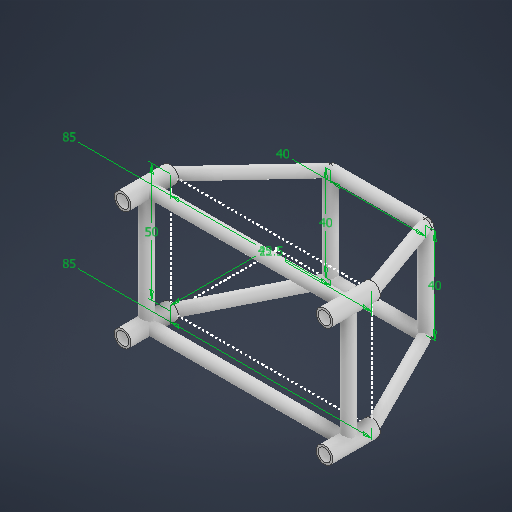
# Autodesk Inventor part: RCPlaneSkeletonFrontFront1
Saved by Autodesk Inventor 2026.1 (Build 301233000, 233)
## iProperties
Created: 2026-03-11
Part Number: RCPlaneSkeletonFrontFront1
Material: Generic
Document SubType Name: Modeling
Designer: morri
Density: 1 g/cm^3
Appearance: Default
Author: morri
Autodesk Inventor part; units mm, degrees
ref_plane "YZ Plane" through (0, 0, 0) normal (1, 0, 0) x (0, 1, 0)
sketch "Sketch1" plane through (0, 0, 0) normal (0, 0, 1) x (1, 0, 0)
  circle A0 centre (0, 0) radius 2.5
  circle A1 centre (0, 50) radius 2.5
  circle A2 centre (85, 50) radius 2.5
  circle A3 centre (85, 0) radius 2.5
  dimension "d10" = 5
  dimension "d11" = 5
  dimension "d12" = 5
  dimension "d13" = 5
  constraints: 4 centre point, 1 coincident
  measures "d10" diameter of A0
  measures "d11" diameter of A1
  measures "d12" diameter of A2
  measures "d13" diameter of A3
sketch3d "3D Sketch1"
  line L0 (85, 50, 0) -> (62.5, 40, -45)
  dimension "d0" = 45
  dimension "d1" = 22.5
  dimension "d2" = 40
  dimension "d3" = 40
  dimension "d4" = 40
  dimension "d5" = 85
  dimension "d6" = 50
  dimension "d7" = 85
sweep "Sweep1" add profiles "Sketch1" path "3D Sketch1" contours A2
sketch3d "3D Sketch1 for Sweep2"
  line L0 (0, 50, 0) -> (22.5, 40, -45)
  dimension "d0" = 45
  dimension "d1" = 22.5
  dimension "d2" = 40
  dimension "d3" = 40
  dimension "d4" = 40
  dimension "d5" = 85
  dimension "d6" = 50
  dimension "d7" = 85
sweep "Sweep2" add profiles "Sketch1" path "3D Sketch1 for Sweep2" separate body contours A1
sketch3d "3D Sketch1 for Sweep3"
  line L0 (0, 0, 0) -> (22.5, 0, -45)
  dimension "d0" = 45
  dimension "d1" = 22.5
  dimension "d2" = 40
  dimension "d3" = 40
  dimension "d4" = 40
  dimension "d5" = 85
  dimension "d6" = 50
  dimension "d7" = 85
sweep "Sweep3" add profiles "Sketch1" path "3D Sketch1 for Sweep3" separate body contours A0
sketch3d "3D Sketch1 for Sweep4"
  line L0 (85, 0, 0) -> (62.5, 0, -45)
  dimension "d0" = 45
  dimension "d1" = 22.5
  dimension "d2" = 40
  dimension "d3" = 40
  dimension "d4" = 40
  dimension "d5" = 85
  dimension "d6" = 50
  dimension "d7" = 85
sweep "Sweep4" add profiles "Sketch1" path "3D Sketch1 for Sweep4" separate body contours A3
ref_plane "Work Plane1" through (0, 0, 0) normal (0, 1, 0) x (-1, 0, 0)
sketch "Sketch2" plane through (0, 0, 0) normal (0, 1, 0) x (-1, 0, 0)
  line L0 (-65, -45) -> (-60, -45) projected
  circle A0 centre (-62.5, -45) radius 2.5
  line L1 (-25, -45) -> (-20, -45) projected
  circle A1 centre (-22.5, -45) radius 2.5
  point P0 (0, 0)
  dimension "d24" = 5
  dimension "d25" = 5
  constraints: 2 centre point, 2 midpoint
  measures "d24" diameter of A0
  measures "d25" diameter of A1
extrude "Extrusion2" add sketch "Sketch2" along normal blind 40 separate body
ref_plane "Work Plane3" through (22.5, 0, -45) normal (-1, 0, 0) x (0, -1, 0)
sketch "Sketch4" plane through (22.5, 0, -45) normal (-1, 0, 0) x (0, -1, 0)
  line L0 (0, 2.5) -> (0, -2.5) projected
  circle A0 centre (0, 0) radius 2.5
  line L1 (-42.5, 0) -> (-37.5, 0) projected
  circle A1 centre (-40, 0) radius 2.5
  point P0 (0, 45)
  dimension "d36" = 5
  dimension "d37" = 5
  constraints: 2 centre point, 2 midpoint
  measures "d36" diameter of A0
  measures "d37" diameter of A1
extrude "Extrusion4" add sketch "Sketch4" against normal blind 40 separate body
sketch "Sketch10" plane through (0, 0, 0) normal (0, 0, 1) x (1, 0, 0)
  circle A0 centre (0, 0) radius 3.5
  circle A1 centre (0, 50) radius 2.5 construction
  circle A2 centre (0, 50) radius 3.5
  circle A3 centre (85, 50) radius 2.5 construction
  circle A4 centre (85, 50) radius 3.5
  circle A5 centre (85, 0) radius 2.5 construction
  circle A6 centre (85, 0) radius 3.5
  dimension "d69" = 7
  dimension "d70" = 7
  dimension "d71" = 7
  dimension "d72" = 7
  constraints: 4 centre point, 4 coincident
  measures "d69" diameter of A0
  measures "d70" diameter of A2
  measures "d71" diameter of A4
  measures "d72" diameter of A6
extrude "Extrusion8" add sketch "Sketch10" along normal blind 20 separate body
sketch "Sketch11" plane through (0, 0, 0) normal (0, 1, 0) x (-1, 0, 0)
  line L0 (0, 0) -> (0, 10) construction
  line L1 (0, 0) -> (-85, 0) construction
  line L2 (-85, 0) -> (-85, 10) construction
  line L3 (-85, 10) -> (0, 10) construction
  line L4 (0, 10) -> (0, 0) construction
  circle A0 centre (0, 10) radius 2.5
  circle A1 centre (-85, 10) radius 2.5
  dimension "d77" = 85
  dimension "d78" = 5
  dimension "d79" = 5
  constraints: 10 end point, 2 centre point, 2 coincident, 2 parallel, 1 horizontal, 1 perpendicular, 1 vertical
  measures "d77" distance of L2.end L3.end
  measures "d78" diameter of A0
  measures "d79" diameter of A1
extrude "Extrusion9" add sketch "Sketch11" along normal blind 50 separate body
sketch "Sketch12" plane through (0, 0, 0) normal (1, 0, 0) x (0, 1, 0)
  circle A0 centre (0, 10) radius 2.5
  line L0 (50, 7.5) -> (50, 12.5) construction
  circle A1 centre (50, 10) radius 2.5
  point P0 (0, 0)
  dimension "d82" = 5
  dimension "d83" = 5
  constraints: 2 centre point, 1 midpoint
  measures "d82" diameter of A0
  measures "d83" diameter of A1
extrude "Extrusion10" add sketch "Sketch12" along normal blind 85 separate body
sketch "Sketch13" plane through (0, 0, 20) normal (0, 0, 1) x (1, 0, 0)
  circle A0 centre (0, 0) radius 2.5 construction
  circle A1 centre (0, 50) radius 2.5 construction
  line L0 (87.5, 50) -> (82.5, 50) construction
  circle A2 centre (85, 0) radius 2.5 construction
  point P0 (85, 50)
  constraints: 3 coincident, 1 midpoint
hole "Hole2" at (0, 0, 20) at (0, 50, 20) at (85, 50, 20) at (85, 0, 20) direction (0, 0, -1) diameter 5.3 depth 15 bodies 7 9 8
equation "\"fitTol\" = 0.3"
body "Solid1"
body "Solid4"
body "Solid5"
body "Solid6"
body "Solid8"
body "Solid10"
body "Solid14"
body "Solid15"
body "Solid16"
